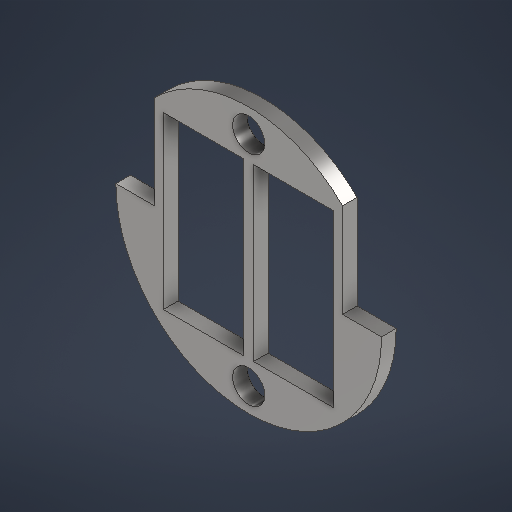
# Autodesk Inventor part: Part3_A_Y
Saved by Autodesk Inventor 2026 (Build 300175050, 175E)
## iProperties
Created: 2026-01-08
Part Number: Part3_A_Y
Material: 鋼、軟鋼
Document SubType Name: Modeling
Designer: Kota-Inoue
Density: 7.85 g/cm^3
Appearance: 半つや出し
Mass: 641.479 g
Surface Area: 319.402 cm^2
Volume: 81.7171 cm^3
Author: Kota-Inoue
Autodesk Inventor part; units mm, degrees
ref_plane "YZ Plane" through (0, 0, 0) normal (1, 0, 0) x (0, 1, 0)
ref_plane "XZ Plane" through (0, 0, 0) normal (0, 1, 0) x (-1, 0, 0)
ref_plane "XY Plane" through (0, 0, 0) normal (0, 0, 1) x (1, 0, 0)
sketch "スケッチ1" plane through (0, 0, 0) normal (0, 0, 1) x (1, 0, 0)
  circle A0 centre (0, 0) radius 27.25
  line L0 (17.5, 17.5) -> (-17.5, 17.5)
  line L1 (-17.5, 17.5) -> (-17.5, -17.5)
  line L2 (-17.5, -17.5) -> (17.5, -17.5)
  line L3 (17.5, -17.5) -> (17.5, 17.5)
  line L4 (17.5, 17.5) -> (-17.5, -17.5) construction
  line L5 (-17.5, 17.5) -> (17.5, -17.5) construction
  line L6 (1, 17.5) -> (-1, 17.5)
  line L7 (-1, 17.5) -> (-1, -17.5)
  line L8 (-1, -17.5) -> (1, -17.5)
  line L9 (1, -17.5) -> (1, 17.5)
  line L10 (1, 17.5) -> (-1, -17.5) construction
  line L11 (-1, 17.5) -> (1, -17.5) construction
  point P0 (1, -17.5)
  point P1 (1, 17.5)
  point P2 (-1, 17.5)
  point P3 (-1, -17.5)
  dimension "d0" = 54.5
  dimension "d6" = 35
  dimension "d107" = 2
  dimension "d108" = 35
  constraints: 24 end point, 4 midpoint, 4 parallel, 3 perpendicular, 2 horizontal, 1 centre point, 1 coincident
  measures "d0" diameter of A0
  measures "d6" distance of L0.start L0.end
  measures "d107" distance of L8.end L7.end
  measures "d108" distance of L7.end L6.end
extrude "押し出し1" add sketch "スケッチ1" against normal blind 3 contours A0 | L9 L2 L7 L0
sketch "スケッチ2" plane through (0, 0, 0) normal (0, 0, 1) x (1, 0, 0)
  line L0 (0, 42.4511) -> (0, -37.5489)
  line L1 (38.0038, 0) -> (-41.9962, 0)
  line L2 (27.25, 42.0143) -> (27.25, -37.9857)
  circle A0 centre (0, 0) radius 27.25 projected
  line L3 (17.5, 17.5) -> (17.5, -17.5) projected
  line L4 (19.25, 25) -> (27.25, 25)
  line L5 (27.25, 25) -> (27.25, -25)
  line L6 (27.25, -25) -> (19.25, -25)
  line L7 (19.25, -25) -> (19.25, 25)
  line L8 (19.25, 25) -> (27.25, -25) construction
  line L9 (27.25, 25) -> (19.25, -25) construction
  point P0 (17.5, 0)
  point P1 (23.25, 0)
  point P2 (19.25, 0)
  point P3 (27.25, 0)
  dimension "d13" = 9.75
  dimension "d14" = 8
  dimension "d15" = 50
  dimension "d19" = 54.5
  dimension "d110" = 1.75
  constraints: 18 end point, 3 midpoint, 3 point on line, 2 horizontal, 2 parallel, 2 vertical, 1 collinear, 1 perpendicular, 1 tangent
  measures "d13" distance from line of L2 point (17.5, 0)
  measures "d14" distance of L5.end L6.end
  measures "d15" distance of L4.end L5.end
  measures "d19" diameter of A0
  measures "d110" distance between parallel lines of L7 L3
extrude "押し出し2" cut sketch "スケッチ2" against normal blind 10 contours L7 L4 L2 A0 | A0 L1 L7 picked at (20.3822, 11.481)
mirror "ミラー1" about plane through (0, 0, 0) normal (1, 0, 0) of "押し出し2"
sketch "スケッチ8" plane through (0, 0, 0) normal (0, 0, 1) x (1, 0, 0)
  circle A0 centre (0, 0) radius 22.375
  circle A1 centre (0, 0) radius 27.25
  line L0 (0, 31.1603) -> (0, -30.8706)
  point P0 (0, 0)
  point P1 (0, 22.375)
  point P2 (0, -22.375)
  dimension "d112" = 44.75
  dimension "d113" = 54.5
  constraints: 2 centre point, 2 coincident, 2 end point, 2 point on circle, 2 point on line, 1 line through centre, 1 vertical
  measures "d112" diameter of A0
  measures "d113" diameter of A1
hole "穴5" at (0, 22.375, 0) at (0, -22.375, 0) direction (0, 0, -1) diameter 6.6 end through all clearance for "Countersunk Flat Head Screw ISO 2009/7046" size "M6" standard "ISO"
